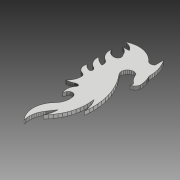
# Autodesk Inventor part: dragon
Saved by Autodesk Inventor 2018 (Build 220112000, 112)
## iProperties
Created: 2019-02-21
Part Number: dragon
Material: 一般
Document SubType Name: Modeling
Designer: ku_sk
Density: 1 g/cm^3
Appearance: 既定
Author: ku_sk
Autodesk Inventor part; units mm, degrees
ref_plane "YZ Plane" through (0, 0, 0) normal (1, 0, 0) x (0, 1, 0)
ref_plane "XZ Plane" through (0, 0, 0) normal (0, 1, 0) x (-1, 0, 0)
ref_plane "XY Plane" through (0, 0, 0) normal (0, 0, 1) x (1, 0, 0)
sketch "スケッチ2" plane through (0, 0, 0) normal (0, 0, 1) x (1, 0, 0)
  line L0 (8.2283, 47.185) -> (8.2963, 47.095) projected
  line L1 (8.2963, 47.095) -> (8.3143, 47.073) projected
  line L2 (8.3143, 47.073) -> (8.3303, 47.049) projected
  line L3 (8.3303, 47.049) -> (8.3643, 47.005) projected
  line L4 (8.3643, 47.005) -> (8.4443, 46.917) projected
  line L5 (8.4443, 46.917) -> (8.5143, 46.839) projected
  line L6 (8.5143, 46.839) -> (8.7603, 46.601) projected
  line L7 (8.7603, 46.601) -> (9.0063, 46.391) projected
  line L8 (9.0063, 46.391) -> (9.2963, 46.175) projected
  line L9 (9.2963, 46.175) -> (9.5183, 46.031) projected
  line L10 (9.5183, 46.031) -> (9.8823, 45.823) projected
  line L11 (9.8823, 45.823) -> (10.1923, 45.677) projected
  line L12 (10.1923, 45.677) -> (10.5103, 45.551) projected
  line L13 (10.5103, 45.551) -> (10.8463, 45.445) projected
  line L14 (10.8463, 45.445) -> (11.1683, 45.365) projected
  line L15 (11.1683, 45.365) -> (11.3043, 45.347) projected
  line L16 (11.3043, 45.347) -> (11.4403, 45.351) projected
  line L17 (11.4403, 45.351) -> (11.5743, 45.377) projected
  line L18 (11.5743, 45.377) -> (11.7023, 45.423) projected
  line L19 (11.7023, 45.423) -> (11.8223, 45.491) projected
  line L20 (11.8223, 45.491) -> (11.9283, 45.575) projected
  line L21 (11.9283, 45.575) -> (12.0203, 45.677) projected
  line L22 (12.0203, 45.677) -> (12.0963, 45.791) projected
  line L23 (12.0963, 45.791) -> (12.1523, 45.915) projected
  line L24 (12.1523, 45.915) -> (12.1863, 46.047) projected
  line L25 (12.1863, 46.047) -> (12.2003, 46.183) projected
  line L26 (12.2003, 46.183) -> (12.1923, 46.321) projected
  line L27 (12.1923, 46.321) -> (12.1943, 46.357) projected
  line L28 (12.1943, 46.357) -> (12.1743, 46.529) projected
  line L29 (12.1743, 46.529) -> (12.1363, 46.697) projected
  line L30 (12.1363, 46.697) -> (12.0823, 46.861) projected
  line L31 (12.0823, 46.861) -> (12.0143, 47.019) projected
  line L32 (12.0143, 47.019) -> (11.9303, 47.171) projected
  line L33 (11.9303, 47.171) -> (11.8323, 47.313) projected
  line L34 (11.8323, 47.313) -> (11.7203, 47.447) projected
  line L35 (11.7203, 47.447) -> (11.5983, 47.567) projected
  line L36 (11.5983, 47.567) -> (11.4643, 47.677) projected
  line L37 (11.4643, 47.677) -> (11.3203, 47.773) projected
  line L38 (11.3203, 47.773) -> (11.1683, 47.855) projected
  line L39 (11.1683, 47.855) -> (10.5903, 48.169) projected
  line L40 (10.5903, 48.169) -> (10.0483, 48.539) projected
  line L41 (10.0483, 48.539) -> (9.5463, 48.965) projected
  line L42 (9.5463, 48.965) -> (9.0923, 49.437) projected
  line L43 (9.0923, 49.437) -> (8.6863, 49.955) projected
  line L44 (8.6863, 49.955) -> (8.3363, 50.511) projected
  line L45 (8.3363, 50.511) -> (8.0463, 51.101) projected
  line L46 (8.0463, 51.101) -> (7.8163, 51.717) projected
  line L47 (7.8163, 51.717) -> (7.6523, 52.353) projected
  line L48 (7.6523, 52.353) -> (7.5523, 53.001) projected
  line L49 (7.5523, 53.001) -> (7.5203, 53.659) projected
  line L50 (7.5203, 53.659) -> (7.5563, 54.315) projected
  line L51 (7.5563, 54.315) -> (7.8723, 53.963) projected
  line L52 (7.8723, 53.963) -> (8.2063, 53.627) projected
  line L53 (8.2063, 53.627) -> (8.5543, 53.307) projected
  line L54 (8.5543, 53.307) -> (8.9183, 53.005) projected
  line L55 (8.9183, 53.005) -> (9.2963, 52.721) projected
  line L56 (9.2963, 52.721) -> (9.6863, 52.453) projected
  line L57 (9.6863, 52.453) -> (10.0883, 52.205) projected
  line L58 (10.0883, 52.205) -> (10.5023, 51.977) projected
  line L59 (10.5023, 51.977) -> (10.9263, 51.767) projected
  line L60 (10.9263, 51.767) -> (11.3603, 51.579) projected
  line L61 (11.3603, 51.579) -> (11.8023, 51.409) projected
  line L62 (11.8023, 51.409) -> (12.2523, 51.263) projected
  line L63 (12.2523, 51.263) -> (12.3243, 51.579) projected
  line L64 (12.3243, 51.579) -> (12.3623, 51.899) projected
  line L65 (12.3623, 51.899) -> (12.3643, 52.223) projected
  line L66 (12.3643, 52.223) -> (12.3303, 52.545) projected
  line L67 (12.3303, 52.545) -> (12.2623, 52.859) projected
  line L68 (12.2623, 52.859) -> (12.1583, 53.165) projected
  line L69 (12.1583, 53.165) -> (12.0203, 53.459) projected
  line L70 (12.0203, 53.459) -> (11.8503, 53.735) projected
  line L71 (11.8503, 53.735) -> (11.6523, 53.989) projected
  line L72 (11.6523, 53.989) -> (11.4263, 54.221) projected
  line L73 (11.4263, 54.221) -> (11.1763, 54.425) projected
  line L74 (11.1763, 54.425) -> (10.9063, 54.601) projected
  line L75 (10.9063, 54.601) -> (10.3223, 54.975) projected
  line L76 (10.3223, 54.975) -> (9.7823, 55.405) projected
  line L77 (9.7823, 55.405) -> (9.2863, 55.887) projected
  line L78 (9.2863, 55.887) -> (8.8423, 56.415) projected
  line L79 (8.8423, 56.415) -> (8.4523, 56.987) projected
  line L80 (8.4523, 56.987) -> (8.1243, 57.595) projected
  line L81 (8.1243, 57.595) -> (7.8583, 58.233) projected
  line L82 (7.8583, 58.233) -> (7.6563, 58.893) projected
  line L83 (7.6563, 58.893) -> (7.5243, 59.571) projected
  line L84 (7.5243, 59.571) -> (7.4603, 60.259) projected
  line L85 (7.4603, 60.259) -> (7.4643, 60.951) projected
  line L86 (7.4643, 60.951) -> (7.5403, 61.637) projected
  line L87 (7.5403, 61.637) -> (7.7063, 61.161) projected
  line L88 (7.7063, 61.161) -> (7.9283, 60.707) projected
  line L89 (7.9283, 60.707) -> (8.1983, 60.281) projected
  line L90 (8.1983, 60.281) -> (8.5163, 59.889) projected
  line L91 (8.5163, 59.889) -> (8.8763, 59.535) projected
  line L92 (8.8763, 59.535) -> (9.2763, 59.225) projected
  line L93 (9.2763, 59.225) -> (9.7063, 58.961) projected
  line L94 (9.7063, 58.961) -> (10.1643, 58.749) projected
  line L95 (10.1643, 58.749) -> (10.6463, 58.591) projected
  line L96 (10.6463, 58.591) -> (11.1403, 58.489) projected
  line L97 (11.1403, 58.489) -> (11.6423, 58.445) projected
  line L98 (11.6423, 58.445) -> (12.1483, 58.457) projected
  line L99 (12.1483, 58.457) -> (12.5203, 58.525) projected
  line L100 (12.5203, 58.525) -> (12.8743, 58.661) projected
  line L101 (12.8743, 58.661) -> (13.1943, 58.865) projected
  line L102 (13.1943, 58.865) -> (13.4703, 59.125) projected
  line L103 (13.4703, 59.125) -> (13.6883, 59.435) projected
  line L104 (13.6883, 59.435) -> (13.8463, 59.779) projected
  line L105 (13.8463, 59.779) -> (13.9323, 60.149) projected
  line L106 (13.9323, 60.149) -> (13.9483, 60.527) projected
  line L107 (13.9483, 60.527) -> (13.8883, 60.901) projected
  line L108 (13.8883, 60.901) -> (13.7603, 61.259) projected
  line L109 (13.7603, 61.259) -> (13.5643, 61.583) projected
  line L110 (13.5643, 61.583) -> (13.3103, 61.863) projected
  line L111 (13.3103, 61.863) -> (13.1083, 62.369) projected
  line L112 (13.1083, 62.369) -> (12.8623, 62.853) projected
  line L113 (12.8623, 62.853) -> (12.5743, 63.313) projected
  line L114 (12.5743, 63.313) -> (12.2443, 63.745) projected
  line L115 (12.2443, 63.745) -> (11.8783, 64.143) projected
  line L116 (11.8783, 64.143) -> (11.4763, 64.509) projected
  line L117 (11.4763, 64.509) -> (11.0443, 64.837) projected
  line L118 (11.0443, 64.837) -> (10.5823, 65.123) projected
  line L119 (10.5823, 65.123) -> (10.0983, 65.367) projected
  line L120 (10.0983, 65.367) -> (9.5923, 65.565) projected
  line L121 (9.5923, 65.565) -> (9.0703, 65.717) projected
  line L122 (9.0703, 65.717) -> (9.1283, 65.747) projected
  line L123 (9.1283, 65.747) -> (9.3303, 65.725) projected
  line L124 (9.3303, 65.725) -> (9.6823, 65.699) projected
  line L125 (9.6823, 65.699) -> (9.7283, 65.695) projected
  line L126 (9.7283, 65.695) -> (10.1263, 65.665) projected
  line L127 (10.1263, 65.665) -> (10.5243, 65.655) projected
  line L128 (10.5243, 65.655) -> (10.9243, 65.645) projected
  line L129 (10.9243, 65.645) -> (11.3223, 65.651) projected
  line L130 (11.3223, 65.651) -> (12.1203, 65.689) projected
  line L131 (12.1203, 65.689) -> (12.9143, 65.769) projected
  line L132 (12.9143, 65.769) -> (12.6183, 66.225) projected
  line L133 (12.6183, 66.225) -> (12.2803, 66.653) projected
  line L134 (12.2803, 66.653) -> (11.9023, 67.047) projected
  line L135 (11.9023, 67.047) -> (11.4903, 67.403) projected
  line L136 (11.4903, 67.403) -> (11.1223, 67.663) projected
  line L137 (11.1223, 67.663) -> (10.5723, 67.989) projected
  line L138 (10.5723, 67.989) -> (10.0763, 68.213) projected
  line L139 (10.0763, 68.213) -> (9.5623, 68.391) projected
  line L140 (9.5623, 68.391) -> (9.0163, 68.521) projected
  line L141 (9.0163, 68.521) -> (8.7543, 68.559) projected
  line L142 (8.7543, 68.559) -> (8.4923, 68.595) projected
  line L143 (8.4923, 68.595) -> (7.9483, 68.621) projected
  line L144 (7.9483, 68.621) -> (7.6703, 68.621) projected
  line L145 (7.6703, 68.621) -> (7.9483, 68.861) projected
  line L146 (7.9483, 68.861) -> (8.7123, 69.239) projected
  line L147 (8.7123, 69.239) -> (10.0823, 69.731) projected
  line L148 (10.0823, 69.731) -> (11.5003, 70.069) projected
  line L149 (11.5003, 70.069) -> (12.9483, 70.243) projected
  line L150 (12.9483, 70.243) -> (14.4063, 70.255) projected
  line L151 (14.4063, 70.255) -> (15.8563, 70.101) projected
  line L152 (15.8563, 70.101) -> (17.2783, 69.787) projected
  line L153 (17.2783, 69.787) -> (17.6123, 69.673) projected
  line L154 (17.6123, 69.673) -> (17.6123, 72.165) projected
  line L155 (17.6123, 72.165) -> (19.0823, 72.165) projected
  line L156 (19.0823, 72.165) -> (19.0823, 69.113) projected
  line L157 (19.0823, 69.113) -> (19.9743, 68.691) projected
  line L158 (19.9743, 68.691) -> (21.2143, 67.923) projected
  line L159 (21.2143, 67.923) -> (22.3583, 67.021) projected
  line L160 (22.3583, 67.021) -> (23.3943, 65.995) projected
  line L161 (23.3943, 65.995) -> (23.6383, 65.761) projected
  line L162 (23.6383, 65.761) -> (23.9103, 65.563) projected
  line L163 (23.9103, 65.563) -> (24.2103, 65.405) projected
  line L164 (24.2103, 65.405) -> (24.5283, 65.289) projected
  line L165 (24.5283, 65.289) -> (24.8583, 65.219) projected
  line L166 (24.8583, 65.219) -> (25.1943, 65.195) projected
  line L167 (25.1943, 65.195) -> (25.5303, 65.219) projected
  line L168 (25.5303, 65.219) -> (25.8623, 65.289) projected
  line L169 (25.8623, 65.289) -> (26.1783, 65.405) projected
  line L170 (26.1783, 65.405) -> (26.4783, 65.563) projected
  line L171 (26.4783, 65.563) -> (26.7503, 65.761) projected
  line L172 (26.7503, 65.761) -> (26.9943, 65.995) projected
  line L173 (26.9943, 65.995) -> (27.0123, 67.543) projected
  line L174 (27.5783, 69.781) -> (27.0123, 67.543) projected
  line L175 (27.8223, 53.223) -> (27.5783, 69.781) projected
  line L176 (28.1303, 52.849) -> (27.8223, 53.223) projected
  line L177 (28.6043, 67.985) -> (28.1303, 52.849) projected
  line L178 (28.115, 68.8963) -> (28.6043, 67.985) projected
  line L179 (28.1124, 68.9005) -> (28.115, 68.8963) projected
  line L180 (27.5783, 69.781) -> (28.1124, 68.9005) projected
  line L181 (26.9943, 70.635) -> (27.5783, 69.781) projected
  line L182 (27.0003, 70.249) -> (26.9943, 70.635) projected
  line L183 (27.0023, 70.113) -> (27.0003, 70.249) projected
  line L184 (27.0023, 69.883) -> (27.0023, 70.113) projected
  line L185 (27.0023, 69.883) -> (27.5783, 69.781) projected
  line L186 (7.9583, 47.539) -> (8.2283, 47.185) projected
  line L187 (7.8803, 47.643) -> (7.9583, 47.539) projected
  line L188 (7.7103, 47.087) -> (7.8803, 47.643) projected
  line L189 (7.6203, 46.511) -> (7.7103, 47.087) projected
  line L190 (7.6103, 45.929) -> (7.6203, 46.511) projected
  line L191 (7.6823, 45.351) -> (7.6103, 45.929) projected
  line L192 (7.8323, 44.789) -> (7.6823, 45.351) projected
  line L193 (8.0603, 44.255) -> (7.8323, 44.789) projected
  line L194 (8.3623, 43.755) -> (8.0603, 44.255) projected
  line L195 (8.7283, 43.303) -> (8.3623, 43.755) projected
  line L196 (9.1543, 42.907) -> (8.7283, 43.303) projected
  line L197 (9.6323, 42.575) -> (9.1543, 42.907) projected
  line L198 (10.1503, 42.311) -> (9.6323, 42.575) projected
  line L199 (10.7023, 42.121) -> (10.1503, 42.311) projected
  line L200 (10.9063, 42.055) -> (10.7023, 42.121) projected
  line L201 (11.1023, 41.967) -> (10.9063, 42.055) projected
  line L202 (11.2863, 41.859) -> (11.1023, 41.967) projected
  line L203 (11.4583, 41.731) -> (11.2863, 41.859) projected
  line L204 (11.6163, 41.585) -> (11.4583, 41.731) projected
  line L205 (11.7583, 41.423) -> (11.6163, 41.585) projected
  line L206 (11.8803, 41.247) -> (11.7583, 41.423) projected
  line L207 (11.9823, 41.059) -> (11.8803, 41.247) projected
  line L208 (12.0663, 40.861) -> (11.9823, 41.059) projected
  line L209 (12.1243, 40.655) -> (12.0663, 40.861) projected
  line L210 (12.1623, 40.443) -> (12.1243, 40.655) projected
  line L211 (12.1763, 40.229) -> (12.1623, 40.443) projected
  line L212 (12.1643, 39.657) -> (12.1763, 40.229) projected
  line L213 (12.1063, 39.089) -> (12.1643, 39.657) projected
  line L214 (12.0083, 38.525) -> (12.1063, 39.089) projected
  line L215 (11.8683, 37.971) -> (12.0083, 38.525) projected
  line L216 (11.6863, 37.429) -> (11.8683, 37.971) projected
  line L217 (11.4643, 36.901) -> (11.6863, 37.429) projected
  line L218 (11.2043, 36.393) -> (11.4643, 36.901) projected
  line L219 (10.9063, 35.905) -> (11.2043, 36.393) projected
  line L220 (10.5723, 35.439) -> (10.9063, 35.905) projected
  line L221 (10.2043, 35.001) -> (10.5723, 35.439) projected
  line L222 (9.8063, 34.593) -> (10.2043, 35.001) projected
  line L223 (9.3763, 34.213) -> (9.8063, 34.593) projected
  line L224 (9.6863, 34.223) -> (9.3763, 34.213) projected
  line L225 (9.9963, 34.243) -> (9.6863, 34.223) projected
  line L226 (10.3043, 34.273) -> (9.9963, 34.243) projected
  line L227 (10.6123, 34.313) -> (10.3043, 34.273) projected
  line L228 (10.9163, 34.365) -> (10.6123, 34.313) projected
  line L229 (11.2203, 34.429) -> (10.9163, 34.365) projected
  line L230 (11.5223, 34.501) -> (11.2203, 34.429) projected
  line L231 (11.8203, 34.585) -> (11.5223, 34.501) projected
  line L232 (12.1163, 34.679) -> (11.8203, 34.585) projected
  line L233 (12.4083, 34.783) -> (12.1163, 34.679) projected
  line L234 (12.6963, 34.897) -> (12.4083, 34.783) projected
  line L235 (13.1183, 35.083) -> (12.6963, 34.897) projected
  line L236 (13.2563, 35.139) -> (13.1183, 35.083) projected
  line L237 (13.3963, 35.195) -> (13.2563, 35.139) projected
  line L238 (13.5383, 35.245) -> (13.3963, 35.195) projected
  line L239 (13.6803, 35.293) -> (13.5383, 35.245) projected
  line L240 (13.8243, 35.337) -> (13.6803, 35.293) projected
  line L241 (13.9703, 35.379) -> (13.8243, 35.337) projected
  line L242 (14.1143, 35.417) -> (13.9703, 35.379) projected
  line L243 (14.2623, 35.451) -> (14.1143, 35.417) projected
  line L244 (14.4083, 35.481) -> (14.2623, 35.451) projected
  line L245 (14.5563, 35.509) -> (14.4083, 35.481) projected
  line L246 (14.7043, 35.535) -> (14.5563, 35.509) projected
  line L247 (14.8823, 35.541) -> (14.7043, 35.535) projected
  line L248 (15.0583, 35.513) -> (14.8823, 35.541) projected
  line L249 (15.2223, 35.447) -> (15.0583, 35.513) projected
  line L250 (15.3703, 35.347) -> (15.2223, 35.447) projected
  line L251 (15.4923, 35.219) -> (15.3703, 35.347) projected
  line L252 (15.5863, 35.069) -> (15.4923, 35.219) projected
  line L253 (15.6443, 34.901) -> (15.5863, 35.069) projected
  line L254 (15.6683, 34.725) -> (15.6443, 34.901) projected
  line L255 (15.6523, 34.549) -> (15.6683, 34.725) projected
  line L256 (15.6023, 34.379) -> (15.6523, 34.549) projected
  line L257 (15.5143, 34.223) -> (15.6023, 34.379) projected
  line L258 (15.3983, 34.091) -> (15.5143, 34.223) projected
  line L259 (15.0463, 33.607) -> (15.3983, 34.091) projected
  line L260 (14.7443, 33.089) -> (15.0463, 33.607) projected
  line L261 (14.4903, 32.547) -> (14.7443, 33.089) projected
  line L262 (14.2903, 31.983) -> (14.4903, 32.547) projected
  line L263 (14.1463, 31.403) -> (14.2903, 31.983) projected
  line L264 (14.0563, 30.811) -> (14.1463, 31.403) projected
  line L265 (14.0243, 30.213) -> (14.0563, 30.811) projected
  line L266 (14.0483, 29.615) -> (14.0243, 30.213) projected
  line L267 (14.1303, 29.021) -> (14.0483, 29.615) projected
  line L268 (14.2683, 28.439) -> (14.1303, 29.021) projected
  line L269 (14.4603, 27.873) -> (14.2683, 28.439) projected
  line L270 (14.7043, 27.327) -> (14.4603, 27.873) projected
  line L271 (15.2963, 28.901) -> (14.7043, 27.327) projected
  line L272 (15.5603, 29.305) -> (15.2963, 28.901) projected
  line L273 (15.9063, 29.641) -> (15.5603, 29.305) projected
  line L274 (16.3163, 29.893) -> (15.9063, 29.641) projected
  line L275 (16.7723, 30.049) -> (16.3163, 29.893) projected
  line L276 (17.2523, 30.103) -> (16.7723, 30.049) projected
  line L277 (17.7303, 30.049) -> (17.2523, 30.103) projected
  line L278 (18.1883, 29.893) -> (17.7303, 30.049) projected
  line L279 (18.5983, 29.641) -> (18.1883, 29.893) projected
  line L280 (18.9443, 29.305) -> (18.5983, 29.641) projected
  line L281 (19.2083, 28.901) -> (18.9443, 29.305) projected
  line L282 (19.3783, 28.449) -> (19.2083, 28.901) projected
  line L283 (19.5263, 27.735) -> (19.3783, 28.449) projected
  line L284 (19.6163, 27.009) -> (19.5263, 27.735) projected
  line L285 (19.6423, 26.279) -> (19.6163, 27.009) projected
  line L286 (19.6063, 25.547) -> (19.6423, 26.279) projected
  line L287 (19.5103, 24.823) -> (19.6063, 25.547) projected
  line L288 (19.3503, 24.109) -> (19.5103, 24.823) projected
  line L289 (19.1323, 23.411) -> (19.3503, 24.109) projected
  line L290 (19.1323, 23.411) -> (19.0463, 13.995) projected
  line L291 (19.0463, 13.995) -> (18.8223, 13.643) projected
  line L292 (18.8223, 13.643) -> (18.5223, 22.085) projected
  line L293 (18.1343, 21.465) -> (18.5223, 22.085) projected
  line L294 (17.6963, 20.879) -> (18.1343, 21.465) projected
  line L295 (17.2103, 20.335) -> (17.6963, 20.879) projected
  line L296 (16.2083, 19.159) -> (17.2103, 20.335) projected
  line L297 (15.3643, 17.867) -> (16.2083, 19.159) projected
  line L298 (14.6923, 16.475) -> (15.3643, 17.867) projected
  line L299 (14.2043, 15.009) -> (14.6923, 16.475) projected
  line L300 (14.2043, 15.009) -> (13.9103, 10.413) projected
  line L301 (14.2043, 8.897) -> (13.9103, 10.413) projected
  line L302 (14.6923, 7.431) -> (14.2043, 8.897) projected
  line L303 (15.3643, 6.041) -> (14.6923, 7.431) projected
  line L304 (16.2083, 4.747) -> (15.3643, 6.041) projected
  line L305 (17.2103, 3.573) -> (16.2083, 4.747) projected
  line L306 (16.9803, 4.423) -> (17.2103, 3.573) projected
  line L307 (16.8143, 5.287) -> (16.9803, 4.423) projected
  line L308 (16.7183, 6.163) -> (16.8143, 5.287) projected
  line L309 (16.6883, 7.043) -> (16.7183, 6.163) projected
  line L310 (16.7243, 7.923) -> (16.6883, 7.043) projected
  line L311 (16.8303, 8.797) -> (16.7243, 7.923) projected
  line L312 (17.0043, 9.661) -> (16.8303, 8.797) projected
  line L313 (17.2423, 10.509) -> (17.0043, 9.661) projected
  line L314 (17.5463, 11.337) -> (17.2423, 10.509) projected
  line L315 (17.9103, 12.137) -> (17.5463, 11.337) projected
  line L316 (18.3383, 12.909) -> (17.9103, 12.137) projected
  line L317 (18.8223, 13.643) -> (18.3383, 12.909) projected
  line L318 (27.0123, 67.543) -> (27.0078, 69.4409) projected
  line L319 (27.0078, 69.4409) -> (27.0078, 69.4438) projected
  line L320 (27.0078, 69.4438) -> (27.0023, 69.883) projected
  line L321 (27.8223, 53.223) -> (27.5323, 53.611) projected
  line L322 (27.5323, 53.611) -> (27.2603, 54.011) projected
  line L323 (27.2603, 54.011) -> (27.0063, 54.425) projected
  line L324 (27.0063, 54.425) -> (26.7743, 54.849) projected
  line L325 (26.7743, 54.849) -> (26.5583, 55.283) projected
  line L326 (26.5583, 55.283) -> (26.3663, 55.727) projected
  line L327 (26.3663, 55.727) -> (26.1923, 56.179) projected
  line L328 (26.1923, 56.179) -> (25.5063, 56.629) projected
  line L329 (25.5063, 56.629) -> (24.7303, 56.895) projected
  line L330 (24.7303, 56.895) -> (23.9143, 56.965) projected
  line L331 (23.9143, 56.965) -> (23.1043, 56.829) projected
  line L332 (23.1043, 56.829) -> (22.3523, 56.499) projected
  line L333 (22.3523, 56.499) -> (21.7043, 55.995) projected
  line L334 (21.7043, 55.995) -> (21.2023, 55.347) projected
  line L335 (21.2023, 55.347) -> (20.8743, 54.595) projected
  line L336 (20.8743, 54.595) -> (20.7403, 53.785) projected
  line L337 (20.7403, 53.785) -> (20.8103, 52.967) projected
  line L338 (20.8103, 52.967) -> (21.0803, 52.193) projected
  line L339 (21.0803, 52.193) -> (21.5303, 51.507) projected
  line L340 (21.5303, 51.507) -> (23.0363, 49.613) projected
  line L341 (23.0363, 49.613) -> (24.4063, 47.619) projected
  line L342 (24.4063, 47.619) -> (25.6343, 45.533) projected
  line L343 (25.6343, 45.533) -> (26.7123, 43.367) projected
  line L344 (26.7123, 43.367) -> (27.6383, 41.131) projected
  line L345 (27.6383, 41.131) -> (28.4043, 38.835) projected
  line L346 (28.4043, 38.835) -> (29.0083, 36.493) projected
  line L347 (29.0083, 36.493) -> (29.4463, 34.113) projected
  line L348 (29.4463, 34.113) -> (29.7183, 31.709) projected
  line L349 (29.7183, 31.709) -> (29.8223, 29.291) projected
  line L350 (29.8223, 29.291) -> (29.7563, 26.871) projected
  line L351 (29.7563, 26.871) -> (29.5223, 24.463) projected
  line L352 (29.5223, 24.463) -> (29.4623, 25.187) projected
  line L353 (29.4623, 25.187) -> (29.3683, 25.907) projected
  line L354 (29.3683, 25.907) -> (29.2423, 26.621) projected
  line L355 (29.2423, 26.621) -> (29.1783, 26.907) projected
  line L356 (29.1783, 26.907) -> (29.0843, 27.329) projected
  line L357 (29.0843, 27.329) -> (28.6683, 28.719) projected
  line L358 (28.6683, 28.719) -> (28.4123, 29.399) projected
  line L359 (28.4123, 29.399) -> (28.1263, 30.067) projected
  line L360 (28.1263, 30.067) -> (27.8083, 30.719) projected
  line L361 (27.8083, 30.719) -> (27.4623, 31.357) projected
  line L362 (27.4623, 31.357) -> (27.0863, 31.977) projected
  line L363 (27.0863, 31.977) -> (26.6803, 32.581) projected
  line L364 (26.6803, 32.581) -> (26.9023, 30.677) projected
  line L365 (26.9023, 30.677) -> (26.9783, 28.761) projected
  line L366 (26.9783, 28.761) -> (26.9063, 26.847) projected
  line L367 (26.9063, 26.847) -> (26.6883, 24.943) projected
  line L368 (26.6883, 24.943) -> (26.3243, 23.061) projected
  line L369 (26.3243, 23.061) -> (25.8163, 21.213) projected
  line L370 (25.8163, 21.213) -> (25.1703, 19.409) projected
  line L371 (25.1703, 19.409) -> (24.3863, 17.659) projected
  line L372 (24.3863, 17.659) -> (23.4723, 15.975) projected
  line L373 (23.4723, 15.975) -> (22.4303, 14.367) projected
  line L374 (22.4303, 14.367) -> (21.2683, 12.843) projected
  line L375 (21.2683, 12.843) -> (19.9943, 11.411) projected
  line L376 (19.9943, 11.411) -> (20.2423, 11.909) projected
  line L377 (20.2423, 11.909) -> (20.4703, 12.415) projected
  line L378 (20.4703, 12.415) -> (20.6763, 12.931) projected
  line L379 (20.6763, 12.931) -> (20.8623, 13.453) projected
  line L380 (20.8623, 13.453) -> (21.0283, 13.983) projected
  line L381 (21.0283, 13.983) -> (21.1703, 14.519) projected
  line L382 (21.1703, 14.519) -> (21.3103, 15.155) projected
  line L383 (21.3103, 15.155) -> (21.3943, 15.609) projected
  line L384 (21.3943, 15.609) -> (21.4703, 16.157) projected
  line L385 (21.4703, 16.157) -> (21.5263, 16.709) projected
  line L386 (21.5263, 16.709) -> (21.5518, 17.1182) projected
  line L387 (21.5518, 17.1182) -> (21.5519, 17.1194) projected
  line L388 (21.5519, 17.1194) -> (21.5723, 17.819) projected
  line L389 (21.5723, 17.819) -> (21.3383, 17.475) projected
  line L390 (21.3383, 17.475) -> (21.1043, 17.129) projected
  line L391 (21.1043, 17.129) -> (20.8723, 16.785) projected
  line L392 (20.8723, 16.785) -> (20.6403, 16.437) projected
  line L393 (20.6403, 16.437) -> (20.4083, 16.091) projected
  line L394 (20.4083, 16.091) -> (20.1803, 15.743) projected
  line L395 (20.1803, 15.743) -> (19.9523, 15.395) projected
  line L396 (19.9523, 15.395) -> (19.7243, 15.045) projected
  line L397 (19.7243, 15.045) -> (19.4963, 14.695) projected
  line L398 (19.4963, 14.695) -> (19.2703, 14.347) projected
  line L399 (19.2703, 14.347) -> (19.0463, 13.995) projected
  line L400 (28.4543, 52.489) -> (28.1303, 52.849) projected
  line L401 (28.7963, 52.147) -> (28.4543, 52.489) projected
  line L402 (29.1523, 51.819) -> (28.7963, 52.147) projected
  line L403 (29.5223, 51.507) -> (29.1523, 51.819) projected
  line L404 (29.6763, 51.363) -> (29.5223, 51.507) projected
  line L405 (29.8083, 51.199) -> (29.6763, 51.363) projected
  line L406 (29.9123, 51.017) -> (29.8083, 51.199) projected
  line L407 (29.9903, 50.821) -> (29.9123, 51.017) projected
  line L408 (30.0363, 50.617) -> (29.9903, 50.821) projected
  line L409 (30.0503, 50.407) -> (30.0363, 50.617) projected
  line L410 (30.0363, 50.197) -> (30.0503, 50.407) projected
  line L411 (29.9903, 49.993) -> (30.0363, 50.197) projected
  line L412 (29.9123, 49.797) -> (29.9903, 49.993) projected
  line L413 (29.8083, 49.615) -> (29.9123, 49.797) projected
  line L414 (29.6763, 49.449) -> (29.8083, 49.615) projected
  line L415 (30.0723, 49.567) -> (29.6763, 49.449) projected
  line L416 (30.4543, 49.725) -> (30.0723, 49.567) projected
  line L417 (30.8163, 49.927) -> (30.4543, 49.725) projected
  line L418 (31.1523, 50.167) -> (30.8163, 49.927) projected
  line L419 (31.4603, 50.443) -> (31.1523, 50.167) projected
  line L420 (31.7343, 50.753) -> (31.4603, 50.443) projected
  line L421 (31.9743, 51.089) -> (31.7343, 50.753) projected
  line L422 (32.1743, 51.451) -> (31.9743, 51.089) projected
  line L423 (32.3323, 51.833) -> (32.1743, 51.451) projected
  line L424 (32.3323, 51.833) -> (32.3603, 53.403) projected
  line L425 (32.2823, 53.985) -> (32.3603, 53.403) projected
  line L426 (32.2823, 53.985) -> (32.3323, 51.833) projected
  line L427 (28.6043, 67.985) -> (29.0423, 67.047) projected
  line L428 (29.0423, 67.047) -> (29.4283, 66.087) projected
  line L429 (29.4283, 66.087) -> (29.7623, 65.109) projected
  line L430 (29.8083, 51.199) -> (29.7623, 65.109) projected
  line L431 (18.8579, 22.7349) -> (19.1323, 23.411) projected
  line L432 (18.8577, 22.7344) -> (18.8579, 22.7349) projected
  line L433 (18.5223, 22.085) -> (18.8577, 22.7344) projected
  line L434 (13.9119, 13.4954) -> (14.2043, 15.009) projected
  line L435 (13.9118, 13.4948) -> (13.9119, 13.4954) projected
  line L436 (13.9118, 13.4947) -> (13.9118, 13.4948) projected
  line L437 (13.9117, 13.4939) -> (13.9118, 13.4947) projected
  line L438 (13.8103, 11.953) -> (13.9117, 13.4939) projected
  line L439 (13.9103, 10.413) -> (13.8103, 11.953) projected
  line L440 (21.5723, 17.819) -> (22.4303, 14.367) projected
  line L441 (22.4303, 14.367) -> (21.5263, 16.709) projected
  line L442 (30.2703, 63.103) -> (30.0503, 50.407) projected
  line L443 (30.2703, 63.103) -> (30.4403, 62.083) projected
  line L444 (30.4403, 62.083) -> (30.5563, 61.055) projected
  line L445 (30.5563, 61.055) -> (30.6163, 60.021) projected
  line L446 (30.6163, 60.021) -> (30.6203, 58.987) projected
  line L447 (30.6203, 58.987) -> (30.8883, 58.463) projected
  line L448 (31.1523, 50.167) -> (30.8883, 58.463) projected
  line L449 (31.3643, 57.387) -> (31.1523, 50.167) projected
  line L450 (31.1349, 57.9284) -> (31.3643, 57.387) projected
  line L451 (31.1348, 57.9287) -> (31.1349, 57.9284) projected
  line L452 (30.8883, 58.463) -> (31.1348, 57.9287) projected
  line L453 (32.1743, 51.451) -> (32.0623, 55.143) projected
  line L454 (32.0623, 55.143) -> (32.1828, 54.565) projected
  line L455 (32.1828, 54.565) -> (32.1828, 54.5649) projected
  line L456 (32.1828, 54.5649) -> (32.1828, 54.5647) projected
  line L457 (32.1828, 54.5647) -> (32.1828, 54.5646) projected
  line L458 (32.1828, 54.5646) -> (32.2823, 53.985) projected
  line L459 (32.4448, 52.2291) -> (32.3323, 51.833) projected
  line L460 (32.4448, 52.2292) -> (32.4448, 52.2291) projected
  line L461 (32.4448, 52.2292) -> (32.4448, 52.2292) projected
  line L462 (32.4448, 52.2295) -> (32.4448, 52.2292) projected
  line L463 (32.4447, 52.2298) -> (32.4448, 52.2295) projected
  line L464 (32.4243, 52.655) -> (32.4447, 52.2298) projected
  line L465 (32.3603, 53.403) -> (32.4243, 52.655) projected
  line L466 (29.7623, 65.109) -> (30.0407, 64.1131) projected
  line L467 (30.0407, 64.1131) -> (30.0408, 64.1126) projected
  line L468 (30.0408, 64.1126) -> (30.2703, 63.103) projected
  line L469 (31.3643, 57.387) -> (31.5703, 56.837) projected
  line L470 (31.5703, 56.837) -> (31.7563, 56.277) projected
  line L471 (31.7563, 56.277) -> (31.9203, 55.713) projected
  line L472 (31.9203, 55.713) -> (32.0623, 55.143) projected
  point P0 (0, 0)
extrude "押し出し1" add sketch "スケッチ2" along normal blind 2
sketch "スケッチ3" plane through (0, 0, 2) normal (0, 0, 1) x (1, 0, 0)
  line L0 (17.6123, 72.165) -> (17.6123, 69.673) projected
  line L1 (19.0823, 72.165) -> (17.6123, 72.165) projected
  line L2 (19.0823, 69.113) -> (19.0823, 72.165) projected
  line L3 (17.6123, 69.673) -> (19.0823, 69.113)
  point P0 (0, 0)
  constraints: 2 end point
extrude "押し出し2" cut sketch "スケッチ3" against normal blind 10
